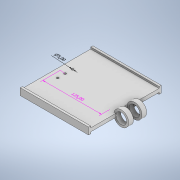
# Autodesk Inventor part: Plataforma deslizante
Saved by Autodesk Inventor 2021 (Build 250183000, 183)
## iProperties
Created: 2021-08-09
Part Number: Plataforma deslizante
Material: Generic
Document SubType Name: Modeling
Designer: guilh
Density: 1 g/cm^3
Appearance: Default
Author: guilh
Autodesk Inventor part; units mm, degrees
ref_plane "YZ Plane" through (0, 0, 0) normal (1, 0, 0) x (0, 1, 0)
ref_plane "XZ Plane" through (0, 0, 0) normal (0, 1, 0) x (-1, 0, 0)
ref_plane "XY Plane" through (0, 0, 0) normal (0, 0, 1) x (1, 0, 0)
sketch "Sketch1" plane through (0, 0, 0) normal (1, 0, 0) x (0, 1, 0)
  line L0 (0, 0) -> (4, 0)
  line L1 (4, 0) -> (4, 80)
  line L2 (4, 80) -> (-4, 80)
  line L3 (-4, 80) -> (-4, -80)
  line L4 (-4, -80) -> (4, -80)
  line L5 (4, -80) -> (4, 0)
  line L6 (4, 80) -> (8, 80)
  line L7 (8, 80) -> (8, 85)
  line L8 (8, 85) -> (-8, 85)
  line L9 (-8, 85) -> (-8, 80)
  line L10 (-8, 80) -> (-4, 80)
  line L11 (-4, -80) -> (-8, -80)
  line L12 (-8, -80) -> (-8, -85)
  line L13 (-8, -85) -> (8, -85)
  line L14 (8, -85) -> (8, -80)
  line L15 (8, -80) -> (4, -80)
  dimension "d0" = 4
  dimension "d1" = 80
  dimension "d2" = 8
  dimension "d3" = 160
  dimension "d4" = 8
  dimension "d5" = 4
  dimension "d6" = 5
  dimension "d7" = 16
  dimension "d8" = 5
  dimension "d9" = 4
  dimension "d10" = 5
  dimension "d11" = 16
  dimension "d12" = 5
  constraints: 32 end point, 7 point on line, 6 perpendicular, 1 collinear, 1 horizontal
  measures "d0" distance of L0.start L0.end
  measures "d1" distance of L0.end L1.end
  measures "d2" distance of L1.end L2.end
  measures "d3" distance of L2.end L3.end
  measures "d4" distance of L3.end L4.end
  measures "d5" distance of L1.end L6.end
  measures "d6" distance of L6.end L7.end
  measures "d7" distance of L7.end L8.end
  measures "d8" distance of L8.end L9.end
  measures "d9" distance of L3.end L11.end
  measures "d10" distance of L11.end L12.end
  measures "d11" distance of L12.end L13.end
  measures "d12" distance of L13.end L14.end
extrude "Extrusion1" add sketch "Sketch1" along normal blind 160
sketch "Sketch2" plane through (0, 4, 80) normal (0, 1, 0) x (1, 0, 0)
  line L0 (0, 160) -> (0, 0) projected
  line L1 (0, 0) -> (0, 80)
  line L2 (0, 80) -> (10, 80)
  circle A0 centre (10, 80) radius 2.5
  line L3 (10, 80) -> (10, 62.5)
  line L4 (10, 80) -> (10, 97.5)
  circle A1 centre (10, 97.5) radius 2.5
  circle A2 centre (10, 62.5) radius 2.5
  dimension "d15" = 80
  dimension "d16" = 10
  dimension "d17" = 5
  dimension "d18" = 17.5
  dimension "d19" = 17.5
  dimension "d20" = 5
  dimension "d21" = 5
  constraints: 8 end point, 3 centre point, 3 coincident, 2 vertical, 1 collinear, 1 perpendicular
  measures "d15" distance of L0.end L1.end
  measures "d16" distance of L1.end L2.end
  measures "d17" diameter of A0
  measures "d18" distance of L3.start L3.end
  measures "d19" distance of L3.start L4.end
  measures "d20" diameter of A1
  measures "d21" diameter of A2
extrude "Extrusion2" cut sketch "Sketch2" against normal blind 10
sketch "Sketch3" plane through (0, 4, 80) normal (0, 1, 0) x (1, 0, 0)
  line L0 (0, 80) -> (20, 80)
  line L1 (20, 80) -> (20, 105.7712)
  line L2 (20, 105.7712) -> (0, 105.7712)
  line L3 (0, 160) -> (0, 0) projected
  line L4 (0, 105.7712) -> (0, 52.2017)
  line L5 (0, 52.2017) -> (20.6954, 52.2017)
  line L6 (20.6954, 52.2017) -> (20, 80)
  dimension "d24" = 20
  constraints: 12 end point, 3 perpendicular, 1 horizontal, 1 point on line, 1 vertical
  measures "d24" distance of L0.start L0.end
extrude "Extrusion3" add sketch "Sketch3" against normal blind 8
sketch "Sketch4" plane through (0, 4, 80) normal (0, 1, 0) x (1, 0, 0)
  line L0 (0, 80) -> (20, 80)
  line L1 (20, 80) -> (20, 97.5)
  line L2 (20, 80) -> (20, 62.5)
  circle A0 centre (20, 97.5) radius 2.5
  circle A1 centre (20, 80) radius 2.5
  circle A2 centre (20, 62.5) radius 2.5
  dimension "d27" = 20
  dimension "d28" = 17.5
  dimension "d29" = 17.5
  dimension "d30" = 5
  dimension "d31" = 5
  dimension "d32" = 5
  constraints: 6 end point, 3 centre point, 3 coincident, 1 horizontal, 1 perpendicular, 1 vertical
  measures "d27" distance of L0.start L0.end
  measures "d28" distance of L0.end L1.end
  measures "d29" distance of L0.end L2.end
  measures "d30" diameter of A0
  measures "d31" diameter of A1
  measures "d32" diameter of A2
extrude "Extrusion4" cut sketch "Sketch4" against normal blind 8
sketch "Sketch5" plane through (0, 4, 80) normal (0, 1, 0) x (1, 0, 0)
  line L0 (0, 80) -> (145, 80)
  line L1 (145, 80) -> (145, 101)
  line L2 (145, 101) -> (160, 101)
  line L3 (160, 0) -> (160, 160) projected
  line L4 (160, 101) -> (160, 59)
  line L5 (160, 59) -> (145, 59)
  line L6 (145, 59) -> (145, 80)
  dimension "d35" = 145
  dimension "d36" = 21
  dimension "d37" = 42
  constraints: 12 end point, 5 perpendicular, 2 point on line, 1 horizontal
  measures "d35" distance of L0.start L0.end
  measures "d36" distance of L0.end L1.end
  measures "d37" distance of L2.end L4.end
extrude "Extrusion5" cut sketch "Sketch5" against normal blind 10
sketch "Sketch6" plane through (0, 4, -80) normal (0, 1, 0) x (1, 0, 0)
  line L0 (0, -80) -> (145, -80)
  line L1 (145, -59) -> (145, -101) projected
  line L2 (145, -80) -> (145, -59)
  line L3 (145, -59) -> (135, -59)
  line L4 (135, -59) -> (135, -99)
  line L5 (135, -99) -> (135, -101)
  line L6 (145, -101) -> (160, -101) projected
  line L7 (135, -101) -> (145, -101)
  line L8 (145, -101) -> (145, -80)
  dimension "d40" = 10
  dimension "d41" = 40
  dimension "d42" = 2
  constraints: 14 end point, 3 perpendicular, 1 midpoint, 1 point on line
  measures "d40" distance of L1.start L3.end
  measures "d41" distance of L3.end L4.end
  measures "d42" distance of L4.end L5.end
extrude "Extrusion6" cut sketch "Sketch6" against normal blind 10
thicken "Thicken1" operation add thickness 10 both sides no extend neighbours yes toward (1, 0, 0) faces at (135, 1.3333, -7)
sketch "Sketch7" plane through (160, -4, -21) normal (0, 0, 1) x (1, 0, 0)
  line L0 (0, 0) -> (-15, 0) projected
  line L1 (-15, 0) -> (2.5, 0)
  line L2 (2.5, 0) -> (2.5, 4)
  line L3 (-14.5367, 0) -> (-15, 0)
  line L4 (-15, 0) -> (-15, 8)
  line L5 (-15, 8) -> (-14.5367, 8)
  line L6 (-15, 8) -> (0, 8) projected
  line L7 (2.5, 4) -> (12.5, 4)
  circle A0 centre (12.5, 4) radius 17.5
  circle A1 centre (12.5, 4) radius 12.5
  line L8 (-14.5367, 8) -> (-4.5367, 8)
  line L9 (-4.5367, 0) -> (-15, 0)
  point P0 (-160, 4)
  point P1 (-4.5367, 0)
  dimension "d51" = 17.5
  dimension "d53" = 4
  dimension "d55" = 10
  dimension "d56" = 25
  constraints: 16 end point, 4 point on line, 2 centre point, 2 collinear, 2 point on circle, 1 coincident, 1 horizontal, 1 parallel, 1 vertical
  measures "d51" distance of L0.end L1.end
  measures "d53" distance of L2.start L2.end
  measures "d55" distance of L7.start L7.end
  measures "d56" diameter of A1
extrude "Extrusion7" add sketch "Sketch7" along normal blind 42
sketch "Sketch8" plane through (0, 4, -80) normal (0, 1, 0) x (1, 0, 0)
  line L0 (160, -59) -> (155.4633, -59) projected
  line L1 (155.4633, -59) -> (155.4633, -70)
  line L2 (155.4633, -70) -> (155.4633, -90)
  line L3 (155.4633, -59) -> (155.4633, -101) projected
  line L4 (155.4633, -90) -> (190, -90)
  line L5 (190, -59) -> (190, -101) projected
  line L6 (190, -90) -> (190, -70)
  line L7 (190, -70) -> (155.4633, -70)
  point P0 (0, -80)
  dimension "d59" = 11
  dimension "d60" = 20
  constraints: 10 end point, 2 perpendicular, 2 point on line, 2 vertical
  measures "d59" distance of L0.end L1.end
  measures "d60" distance of L1.end L2.end
extrude "Extrusion8" cut sketch "Sketch8" along normal mid plane 50
body "Solid1"
